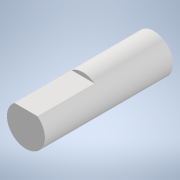
# Autodesk Inventor part: motor_shaft
Saved by Autodesk Inventor 2020 (Build 240168000, 168)
## iProperties
Created: 2020-07-27
Part Number: motor_shaft
Material: Generic
Document SubType Name: Modeling
Designer: Ashiqrahman
Density: 1 g/cm^3
Appearance: Default
Author: Ashiqrahman
Autodesk Inventor part; units mm, degrees
ref_plane "YZ Plane" through (0, 0, 0) normal (1, 0, 0) x (0, 1, 0)
ref_plane "XZ Plane" through (0, 0, 0) normal (0, 1, 0) x (-1, 0, 0)
ref_plane "XY Plane" through (0, 0, 0) normal (0, 0, 1) x (1, 0, 0)
sketch "Sketch1" plane through (0, 0, 0) normal (0, 0, 1) x (1, 0, 0)
  circle A0 centre (0, 0) radius 4
  dimension "d0" = 8
  constraints: 1 centre point, 1 coincident
  measures "d0" diameter of A0
extrude "Extrusion1" add sketch "Sketch1" along normal blind 27
sketch "Sketch2" plane through (0, 0, 27) normal (0, 0, 1) x (1, 0, 0)
  circle A0 centre (0, 0) radius 4 projected
  circle A1 centre (0, 0) radius 4 projected
  line L0 (-2.433, 3.175) -> (2.433, 3.175)
  constraints: 2 end point, 2 point on circle, 1 horizontal
extrude "Extrusion2" cut sketch "Sketch2" against normal blind 12 contours L0 A0 picked at (-0.563, 3.3253)
body "Solid1"
